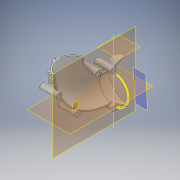
# Autodesk Inventor part: conduit_bis
Saved by Autodesk Inventor 2017 (Build 210142000, 142)
## iProperties
Part Number: conduit_bis
Material: Générique
Document SubType Name: Modeling
Designer: Thomas
Density: 1 g/cm^3
Appearance: Par défaut
Author: Thomas
Autodesk Inventor part; units mm, degrees
ref_plane "XZ Plane" through (0, 0, 0) normal (0, 1, 0) x (-1, 0, 0)
sketch "Esquisse1" plane through (0, 0, 0) normal (0, 0, 1) x (1, 0, 0)
  point P0 (0, 0)
sketch "Esquisse2" plane through (0, 0, 0) normal (0, 1, 0) x (-1, 0, 0)
  line L0 (-7.5, -30.360188) -> (-7.5, 30.360188) construction
  line L1 (-7.5, 30.360188) -> (7.5, 30.360188) construction
  line L2 (7.5, 30.360188) -> (7.5, -30.360188) construction
  line L3 (7.5, -30.360188) -> (-7.5, -30.360188) construction
  arc A0 (-5.995616, 24.270406) -> (-5.995616, -24.270406) centre (0, 0) ccw construction
  arc A1 (-5.995616, 24.270406) -> (-5.995616, -24.270406) centre (0, 0) ccw
  line L4 (-5.995616, -24.270406) -> (-5.995616, -26.325892)
  line L5 (-5.995616, 24.270406) -> (-5.995616, 26.325892)
  arc A2 (-5.995616, 26.325892) -> (-5.995616, -26.325892) centre (0, 0) ccw
  line L6 (-7.5, 30.360188) -> (-5.995616, 24.270406) construction
  dimension "d1" = 15
  constraints: 14 end point, 6 point on circle, 3 centre point, 3 coincident, 3 vertical, 2 parallel, 1 perpendicular
  measures "d1" distance of L0.end L1.end
ref_plane "Plan de construction1" through (0, 0, 70) normal (0, 0, 1) x (1, 0, 0)
sketch "Esquisse3" plane through (0, 0, 70) normal (0, 0, 1) x (1, 0, 0)
  line L0 (0, 0) -> (0, -75) construction
  line L1 (-7.5, -102.5) -> (-7.5, -47.5) construction
  line L2 (-7.5, -47.5) -> (7.5, -47.5) construction
  line L3 (7.5, -47.5) -> (7.5, -102.5) construction
  line L4 (7.5, -102.5) -> (0, -102.5) construction
  line L5 (-7.5, -102.5) -> (7.5, -47.5) construction
  line L6 (-7.5, -47.5) -> (7.5, -102.5) construction
  arc A0 (-7.5, -98.84848) -> (-6.577935, -99.119096) centre (0, -75) ccw
  arc A1 (-7.5, -101.457513) -> (-7.235729, -101.531005) centre (0, -75) ccw
  arc A2 (7.5, -101.457513) -> (7.5, -48.542487) centre (0, -75) ccw
  arc A3 (-7.235729, -48.468995) -> (-7.5, -48.542487) centre (0, -75) ccw
  arc A4 (7.5, -98.84848) -> (7.5, -51.15152) centre (0, -75) ccw
  line L7 (7.5, -48.542487) -> (7.5, -51.15152)
  line L8 (7.5, -98.84848) -> (7.5, -101.457513)
  dimension "d4" = 75
  dimension "d7" = 15
  constraints: 18 end point, 10 point on circle, 10 point on line, 5 centre point, 2 coincident, 2 collinear, 2 midpoint, 2 parallel, 1 perpendicular, 1 vertical
  measures "d4" distance of L0.start L0.end
  measures "d7" distance of L1.end L2.end
sketch "Esquisse4" plane through (0, 0, 0) normal (1, 0, 0) x (0, 1, 0)
  point P0 (0, 0)
ref_plane "Plan de construction2" through (0, 30.375677, -6.052284) normal (0, 0.9985089, 0.0545884) x (1, 0, 0)
sketch "Esquisse6" plane through (0, 30.375677, -6.052284) normal (0, 0.9985089, 0.0545884) x (1, 0, 0)
  line L0 (-7.5, -42) -> (-7.5, 42) construction
  line L1 (-7.5, 42) -> (0, 42) construction
  line L2 (7.5, 42) -> (7.5, -42) construction
  line L3 (7.5, -42) -> (-7.5, -42) construction
  line L4 (-7.5, -42) -> (7.5, 42) construction
  line L5 (-7.5, 42) -> (7.5, -42) construction
  line L6 (7.5, 41.324932) -> (7.5, 39.290584)
  line L7 (7.5, -83.529142) -> (7.5, -23.84848)
  line L8 (7.5, -39.290584) -> (7.5, -41.324932)
  arc A0 (7.5, -39.290584) -> (7.5, 39.290584) centre (0, 0) ccw
  arc A1 (7.5, -41.324932) -> (7.5, 41.324932) centre (0, 0) ccw
  point P0 (0, -7.70142)
  dimension "d13" = 15
  constraints: 16 end point, 6 point on line, 4 point on circle, 2 centre point, 2 midpoint, 2 parallel, 1 coincident, 1 perpendicular, 1 vertical
  measures "d13" distance of L0.end L2.start
sketch "Esquisse7" plane through (0, 0, 0) normal (1, 0, 0) x (0, 1, 0)
  line L0 (0, 0) -> (-75, 0) construction
  line L1 (-75, 0) -> (-75, 70) construction
  line L2 (-75, 70) -> (0, 70) construction
  line L3 (0, 70) -> (0, 0) construction
  line L4 (0, 0) -> (-75, 70) construction
  line L5 (0, 70) -> (-75, 0) construction
  arc A0 (-75, 70) -> (0, 0) centre (0, 75.178571) ccw
  dimension "d18" = 75
  dimension "d19" = 70
  constraints: 12 end point, 2 parallel, 2 point on circle, 1 centre point, 1 horizontal, 1 perpendicular, 1 tangent
  measures "d18" distance of L1.end L2.end
  measures "d19" distance of L0.end L1.end
sweep "Balayage2" add profiles "Esquisse2" path "Esquisse7"
sketch "Esquisse8" plane through (0, 0, 0) normal (0, 1, 0) x (1, 0, 0)
  arc A0 (5.995616, -24.270406) -> (5.995616, 24.270406) centre (0, 0) ccw
  line L0 (5.995616, -24.270406) -> (5.995616, -26.325892)
  arc A1 (5.995616, -26.325892) -> (5.995616, 26.325892) centre (0, 0) ccw
  line L1 (5.995616, 26.325892) -> (5.995616, 24.270406)
loft "Lissage2" add profiles "Esquisse6" section 2 edges at (25, 0, 0) (5.995616, 0, 25.298149) (27, 0, 0) (5.995616, 0, -25.298149)
sketch "Esquisse9" plane through (0, 0, 0) normal (1, 0, 0) x (0, 1, 0)
  circle A0 centre (2.375523, -30.725539) radius 2.25
  circle A1 centre (-64.527837, -6.249705) radius 2.25
  circle A2 centre (-0.329385, 28.911016) radius 2.25
  circle A3 centre (-27.239949, 37.512098) radius 2.25
  circle A4 centre (-97.392349, 38.176402) radius 2.25
  line L0 (32.63154, -47.315598) -> (32.520488, -45.284283)
  line L1 (32.63154, -47.315598) -> (0, -26.325892)
  line L2 (0, -26.325892) -> (0, -24.270406)
  line L3 (32.520488, -45.284283) -> (0, -24.270406)
  line L4 (0, -26.325892) -> (0, -24.270406)
  arc A5 (-101.26336, 68.186578) -> (0, -26.325892) centre (0, 75.178571) ccw
  line L5 (-99.212756, 68.328167) -> (-101.26336, 68.186578)
  arc A6 (-99.212756, 68.328167) -> (0, -24.270406) centre (0, 75.178571) ccw
  line L6 (0, 24.270406) -> (0, 26.325892)
  arc A7 (-50.787244, 71.671833) -> (0, 24.270406) centre (0, 75.178571) ccw
  line L7 (-48.73664, 71.813422) -> (-50.787244, 71.671833)
  arc A8 (-48.73664, 71.813422) -> (0, 26.325892) centre (0, 75.178571) ccw
  line L8 (28.230865, 33.179716) -> (28.119814, 35.21103)
  line L9 (28.230865, 33.179716) -> (0, 24.270406)
  line L10 (0, 24.270406) -> (0, 26.325892)
  line L11 (28.119814, 35.21103) -> (0, 26.325892)
  arc A9 (0, -26.325892) -> (7.364139, -31.062754) centre (2.375523, -30.725539) ccw
  arc A10 (-66.385524, -1.607614) -> (-59.584063, -6.997432) centre (-64.527837, -6.249705) ccw
  arc A11 (4.536137, 27.759194) -> (-4.740264, 26.556414) centre (-0.329385, 28.911016) ccw
  arc A12 (-24.851689, 33.119353) -> (-32.159683, 38.404409) centre (-27.239949, 37.512098) ccw
  arc A13 (-96.286424, 43.052561) -> (-93.327602, 35.26473) centre (-97.392349, 38.176402) ccw
  line L12 (32.63154, -47.315598) -> (0, -26.325892)
  line L13 (7.364139, -31.062754) -> (0, -26.325892)
  line L14 (0, -26.325892) -> (0, -26.325892)
  arc A14 (-101.26336, 68.186578) -> (0, -26.325892) centre (0, 75.178571) ccw
  line L15 (28.119814, 35.21103) -> (0, 26.325892)
  line L16 (4.536137, 27.759194) -> (0, 26.325892)
  line L17 (0, 26.325892) -> (-4.740264, 26.556414)
  arc A15 (-48.73664, 71.813422) -> (0, 26.325892) centre (0, 75.178571) ccw
  arc A16 (-32.159683, 38.404409) -> (-24.851689, 33.119353) centre (0, 75.178571) ccw
  arc A17 (-66.385524, -1.607614) -> (-59.584063, -6.997432) centre (0, 75.178571) ccw
  arc A18 (-96.286424, 43.052561) -> (-93.327602, 35.26473) centre (0, 75.178571) ccw
  point P0 (0, 0)
  dimension "d26" = 4.5
  dimension "d27" = 4.5
  dimension "d28" = 4.5
  dimension "d29" = 4.5
  dimension "d30" = 4.5
  dimension "d31" = 10
  dimension "d32" = 10
  dimension "d33" = 10
  dimension "d34" = 10
  dimension "d35" = 10
  constraints: 24 point on circle, 13 centre point, 8 end point, 5 coincident, 2 collinear, 2 point on line, 1 horizontal, 1 tangent
  measures "d26" diameter of A0
  measures "d27" diameter of A1
  measures "d28" diameter of A2
  measures "d29" diameter of A3
  measures "d30" diameter of A4
  measures "d31" diameter of A9
  measures "d32" diameter of A10
  measures "d33" diameter of A11
  measures "d34" diameter of A12
  measures "d35" diameter of A13
extrude "Extrusion1" add sketch "Esquisse9" along normal blind 30 contours A9 L1 | A10 A5 | A5 A13 | L17 A11 L11 | A8 A12
ref_plane "Plan de construction3" through (30, 0, 0) normal (1, 0, 0) x (0, 0, -1)
sketch "Esquisse10" plane through (30, 0, 0) normal (1, 0, 0) x (0, 0, -1)
  line L0 (-71.813422, -48.73664) -> (-68.186578, -101.26336)
  line L1 (-35.21103, 28.119814) -> (-27.759194, 4.536137)
  arc A0 (-71.813422, -48.73664) -> (-35.21103, 28.119814) centre (-98.225515, 10.986004) ccw
  line L2 (47.315598, 32.63154) -> (31.062754, 7.364139)
  arc A1 (-68.152336, -101.30015) -> (47.315598, 32.63154) centre (-49.477554, -0.6598) ccw
  arc A2 (26.325892, 0) -> (31.062754, 7.364139) centre (30.725539, 2.375523) ccw
  arc A3 (1.607614, -66.385524) -> (6.997432, -59.584063) centre (6.249705, -64.527837) ccw
  arc A4 (-43.052561, -96.286424) -> (-35.26473, -93.327602) centre (-38.176402, -97.392349) ccw
  arc A5 (-33.119353, -24.851689) -> (-38.404409, -32.159683) centre (-37.512098, -27.239949) ccw
  arc A6 (-27.759194, 4.536137) -> (-26.556414, -4.740264) centre (-28.911016, -0.329385) ccw
  arc A7 (-33.119353, -24.851689) -> (-26.556414, -4.740264) centre (-75.178571, 0) ccw
  arc A8 (6.997432, -59.584063) -> (26.325892, 0) centre (-75.178571, 0) ccw
  arc A9 (-35.26473, -93.327602) -> (1.607614, -66.385524) centre (-75.178571, 0) ccw
  arc A10 (-68.186578, -101.26336) -> (-43.052561, -96.286424) centre (-75.178571, 0) ccw
  line L3 (47.315598, 32.63154) -> (-35.21103, 28.119814)
  circle A11 centre (-28.911016, -0.329385) radius 5
  circle A12 centre (-37.512098, -27.239949) radius 5
  circle A13 centre (-38.176402, -97.392349) radius 2.25
  circle A14 centre (-38.176402, -97.392349) radius 5
  circle A15 centre (6.249705, -64.527837) radius 2.25
  circle A16 centre (6.249705, -64.527837) radius 5
  circle A17 centre (30.725539, 2.375523) radius 5
  circle A18 centre (-37.512098, -27.239949) radius 2.25
  circle A19 centre (-28.911016, -0.329385) radius 2.25
  circle A20 centre (30.725539, 2.375523) radius 2.25
  point P0 (0, 0)
  constraints: 7 centre point, 5 coincident, 5 concentric, 4 point on circle
extrude "Extrusion3" add sketch "Esquisse10" against normal blind 30 contours A6 A0 | A0 A6 A11 | A14 A4 A1 | A1 A4 | A16 A3 | A2 A17 | A12 A5
sketch "Esquisse11" plane through (0, -75, 70) normal (0, -0.0688836, 0.9976247) x (1, 0, 0)
  line L0 (0, -29.531285) -> (0, -19.531285)
  arc A0 (5.995616, -24.270406) -> (5.995616, 24.270406) centre (0, 0) ccw
  line L1 (5.995616, -24.270406) -> (5.995616, -26.325892)
  arc A1 (5.995616, -26.325892) -> (5.995616, 26.325892) centre (0, 0) ccw
  line L2 (5.995616, 26.325892) -> (5.995616, 24.270406)
  circle A2 centre (29.233341, 0) radius 1.25
  circle A3 centre (15, -24.879426) radius 1.25
  arc A4 (5.995616, -26.325892) -> (5.995616, 26.325892) centre (0, 0) ccw
  arc A5 (5.995616, -26.325892) -> (5.995616, 26.325892) centre (0, 0) ccw
  arc A6 (25.934098, -7.511496) -> (26.303764, 6.091963) centre (24.028779, -0.652968) ccw
  arc A7 (9.580185, -25.243218) -> (18.174088, -19.967537) centre (13.848884, -22.559355) ccw
  point P0 (0, 70)
  point P1 (2.921341, -2.524646)
  dimension "d43" = 2.5
  dimension "d44" = 2.5
  constraints: 14 point on circle, 5 centre point, 1 concentric
  measures "d43" diameter of A2
  measures "d44" diameter of A3
extrude "Extrusion4" add sketch "Esquisse11" against normal blind 15 contours A1 A7 | A6 A1
mirror "Symétrie1" about plane through (0, 0, 0) normal (1, 0, 0)
sketch "Esquisse12" plane through (0, 0, 0) normal (0, 0, 1) x (1, 0, 0)
  line L0 (0, 38.536351) -> (45.973191, 38.536351)
  line L1 (45.973191, 38.536351) -> (45.973191, -108.510251)
  line L2 (45.973191, -108.510251) -> (0, -108.510251)
  line L3 (0, -108.510251) -> (0, 38.536351)
  point P0 (0, 0)
  constraints: 8 end point, 2 parallel, 1 horizontal, 1 perpendicular
extrude "Extrusion5" cut sketch "Esquisse12" along normal mid plane 206.5
